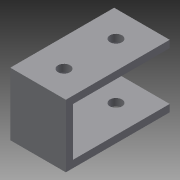
# Autodesk Inventor part: west coast corner
Saved by Autodesk Inventor 2013 (Build 170138000, 138)
## iProperties
Created: 2014-08-13
Part Number: west coast corner
Material: Generic
Document SubType Name: Modeling
Designer: kahohbein
Density: 1 g/cm^3
Author: kahohbein
Autodesk Inventor part; units mm, degrees
ref_plane "YZ Plane" through (0, 0, 0) normal (1, 0, 0) x (0, 1, 0)
ref_plane "XZ Plane" through (0, 0, 0) normal (0, 1, 0) x (-1, 0, 0)
ref_plane "XY Plane" through (0, 0, 0) normal (0, 0, 1) x (1, 0, 0)
sketch "Sketch1" plane through (0, 0, 0) normal (0, 0, 1) x (1, 0, 0)
  line L0 (-12.7, -12.7) -> (12.7, -12.7)
  line L1 (12.7, 12.7) -> (-12.7, 12.7)
  line L2 (-12.7, 12.7) -> (-12.7, -12.7)
  line L3 (-12.7, -12.7) -> (12.7, 12.7) construction
  line L4 (12.7, -12.7) -> (-12.7, 12.7) construction
  line L5 (12.7, 12.7) -> (12.7, 16.51)
  line L6 (12.7, 16.51) -> (-16.51, 16.51)
  line L7 (-16.51, 16.51) -> (-16.51, 12.7)
  line L8 (12.7, -12.7) -> (12.7, -16.51)
  line L9 (12.7, -16.51) -> (-16.51, -16.51)
  line L10 (-16.51, -16.51) -> (-16.51, 12.7)
  point P0 (0, 0)
  dimension "d0" = 25.4
  dimension "d1" = 25.4
  dimension "d2" = 3.81
  dimension "d3" = 29.21
  dimension "d4" = 3.81
  dimension "d5" = 29.21
  constraints: 22 end point, 4 parallel, 2 midpoint, 2 perpendicular, 1 horizontal
  measures "d0" distance of L1.end L1.start
  measures "d1" distance of L1.start L0.end
  measures "d2" distance of L1.start L5.end
  measures "d3" distance of L5.end L6.end
  measures "d4" distance of L0.end L8.end
  measures "d5" distance of L8.end L9.end
extrude "Extrusion1" add sketch "Sketch1" along normal blind 29.21
sketch "Sketch2" plane through (0, 0, 29.21) normal (0, 0, 1) x (1, 0, 0)
  line L0 (12.7, 12.7) -> (12.7, 16.51) projected
  line L1 (12.7, 16.51) -> (-16.51, 16.51) projected
  line L2 (-16.51, 16.51) -> (-16.51, -16.51) projected
  line L3 (-16.51, -16.51) -> (12.7, -16.51) projected
  line L4 (12.7, -16.51) -> (12.7, -12.7) projected
  line L5 (12.7, 12.7) -> (12.7, -12.7)
  point P0 (0, 0)
  constraints: 2 end point, 1 collinear
extrude "Extrusion2" add sketch "Sketch2" against normal blind 3.81
sketch "Sketch3" plane through (0, 0, 0) normal (0, 0, -1) x (-1, 0, 0)
  line L0 (12.7, -12.7) -> (-12.7, -12.7) projected
  line L1 (-12.7, -12.7) -> (-12.7, -16.51) projected
  line L2 (-12.7, -16.51) -> (16.51, -16.51) projected
  line L3 (16.51, -16.51) -> (16.51, 16.51) projected
  line L4 (16.51, 16.51) -> (-12.7, 16.51) projected
  line L5 (-12.7, 16.51) -> (-12.7, 12.7) projected
  line L6 (-12.7, 12.7) -> (12.7, 12.7) projected
  line L7 (12.7, 12.7) -> (12.7, -12.7) projected
  point P0 (0, 0)
extrude "Extrusion3" add sketch "Sketch3" along normal blind 25.4
sketch "Sketch4" plane through (-16.51, 16.51, 29.21) normal (0, 1, 0) x (1, 0, 0)
  circle A0 centre (14.605, 40.9575) radius 3.175
  circle A1 centre (14.605, 13.6525) radius 3.175
  point P0 (16.51, 29.21)
  dimension "d12" = 6.35
  dimension "d13" = 6.35
  constraints: 2 centre point
  measures "d12" diameter of A0
  measures "d13" diameter of A1
extrude "Extrusion4" cut sketch "Sketch4" against normal blind 50.8
body "Solid1"
